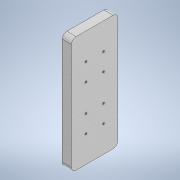
# Autodesk Inventor part: Gehäuse festigung platte
Saved by Autodesk Inventor 2022 (Build 260153000, 153)
## iProperties
Created: 2023-01-30
Part Number: Gehäuse festigung platte
Material: Aluminium 6061
Document SubType Name: Modeling
Designer: Matias Nicky
Density: 2.7 g/cm^3
Appearance: Aluminiumguss
Author: Matias Nicky
Autodesk Inventor part; units mm, degrees
ref_plane "YZ Plane" through (0, 0, 0) normal (1, 0, 0) x (0, 1, 0)
ref_plane "XZ Plane" through (0, 0, 0) normal (0, 1, 0) x (-1, 0, 0)
ref_plane "XY Plane" through (0, 0, 0) normal (0, 0, 1) x (1, 0, 0)
sketch "Skizze1" plane through (0, 0, 0) normal (1, 0, 0) x (0, 1, 0)
  line L0 (-125, 50) -> (125, 50)
  line L1 (125, 50) -> (125, -50)
  line L2 (125, -50) -> (-125, -50)
  line L3 (-125, -50) -> (-125, 50)
  line L4 (-125, 50) -> (125, -50) construction
  line L5 (125, 50) -> (-125, -50) construction
  point P0 (0, 0)
  dimension "d0" = 250
  dimension "d1" = 100
  constraints: 12 end point, 2 midpoint, 2 parallel, 1 horizontal, 1 perpendicular
  measures "d0" distance of L1.end L2.end
  measures "d1" distance between parallel lines of L2 L0
extrude "Extrusion1" add sketch "Skizze1" along normal blind 20
sketch "Skizze2" plane through (20, 0, 0) normal (1, 0, 0) x (0, 0, -1)
  line L0 (25, -23.5) -> (-25, -23.5)
  line L1 (-25, -23.5) -> (-25, -73.5)
  line L2 (-25, -73.5) -> (25, -73.5)
  line L3 (25, -73.5) -> (25, -23.5)
  line L4 (25, -23.5) -> (-25, -73.5) construction
  line L5 (-25, -23.5) -> (25, -73.5) construction
  line L6 (25, 73.5) -> (-25, 73.5)
  line L7 (-25, 73.5) -> (-25, 23.5)
  line L8 (-25, 23.5) -> (25, 23.5)
  line L9 (25, 23.5) -> (25, 73.5)
  line L10 (25, 73.5) -> (-25, 23.5) construction
  line L11 (-25, 73.5) -> (25, 23.5) construction
  point P0 (0, 0)
  point P1 (0, -48.5)
  point P2 (0, 48.5)
  point P3 (-19, -67.5)
  point P4 (-19, -29.5)
  point P5 (19, -29.5)
  point P6 (19, -67.5)
  point P7 (19, 29.5)
  point P8 (19, 67.5)
  point P9 (-19, 67.5)
  point P10 (-19, 29.5)
  dimension "d4" = 50
  dimension "d5" = 50
  dimension "d6" = 50
  dimension "d7" = 50
  dimension "d8" = 97
  dimension "d10" = 48.5
  dimension "d11" = 0
  dimension "d13" = 6
  dimension "d14" = 6
  dimension "d15" = 6
  dimension "d16" = 6
  dimension "d17" = 6
  dimension "d18" = 6
  dimension "d19" = 6
  dimension "d20" = 6
  constraints: 24 end point, 8 point on line, 4 midpoint, 4 parallel, 2 horizontal, 2 perpendicular
  measures "d4" distance of L2.end L1.end
  measures "d5" distance of L1.end L0.end
  measures "d6" distance of L8.end L7.end
  measures "d7" distance of L7.end L6.end
  measures "d8" distance of point (0, 48.5) point (0, -48.5)
  measures "d10" distance of point (0, 0) point (0, -48.5)
  measures "d11" horizontal distance of point (0, 0) point (0, -48.5)
  measures "d13" distance from line of L7 point (-19, 29.5)
  measures "d14" distance from line of L7 point (-19, 67.5)
  measures "d15" distance from line of L9 point (19, 67.5)
  measures "d16" distance from line of L9 point (19, 29.5)
  measures "d17" distance from line of L3 point (19, -29.5)
  measures "d18" distance from line of L1 point (-19, -29.5)
  measures "d19" distance from line of L1 point (-19, -67.5)
  measures "d20" distance from line of L3 point (19, -67.5)
fillet "Rundung1" radius 10 4 edges at (10, -125, 50) (10, -125, -50) (10, 125, -50) (10, 125, 50)
hole "Bohrung1" at (20, -67.5, 19) at (20, -29.5, 19) at (20, -29.5, -19) at (20, -67.5, -19) at (20, 29.5, -19) at (20, 67.5, -19) at (20, 67.5, 19) at (20, 29.5, 19) direction (-1, 0, 0) diameter 4.134 depth 14.2 thread size "M5x0.8" class "6H" standard "ANSI Metric M Profile"
equation "\"d22\" = d19"
